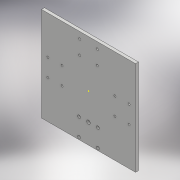
# Autodesk Inventor part: 内层板
Saved by Autodesk Inventor 2017 (Build 210142000, 142)
## iProperties
Part Number: 内层板
Material: 常规
Document SubType Name: 钣金
Designer: PANDA
Density: 1 g/cm^3
Sheet Metal Rule: 默认_mm
Appearance: 默认
Author: PANDA
Autodesk Inventor part; units mm, degrees
ref_plane "YZ Plane" through (0, 0, 0) normal (1, 0, 0) x (0, 1, 0)
ref_plane "XZ Plane" through (0, 0, 0) normal (0, 1, 0) x (-1, 0, 0)
ref_plane "XY Plane" through (0, 0, 0) normal (0, 0, 1) x (1, 0, 0)
sketch "草图19" plane through (0, 0, 0) normal (0, 1, 0) x (-1, 0, 0)
  line L0 (-80, 80) -> (80, 80)
  line L1 (80, 80) -> (80, -80)
  line L2 (80, -80) -> (-80, -80)
  line L3 (-80, -80) -> (-80, 80)
  point P0 (0, 0)
  dimension "d55" = 160
  dimension "d56" = 160
  constraints: 8 end point, 2 parallel, 1 horizontal, 1 perpendicular
  measures "d55" distance of L1.end L2.end
  measures "d56" distance of L0.end L1.end
extrude "拉伸19" add sketch "草图19" along normal blind 5
sketch "草图20" plane through (0, 5, 0) normal (0, 1, 0) x (1, 0, 0)
  circle A0 centre (15, -69) radius 1.8
  point P0 (0, 0)
  dimension "d59" = 3.6
  constraints: 1 centre point
  measures "d59" diameter of A0
extrude "拉伸20" cut sketch "草图20" against normal through all
sketch "草图21" plane through (0, 0, 0) normal (0, -1, 0) x (1, 0, 0)
  circle A0 centre (-15, 69) radius 1.8
  point P0 (0, 0)
  dimension "d62" = 3.6
  constraints: 1 centre point
  measures "d62" diameter of A0
extrude "拉伸21" cut sketch "草图21" against normal through all
sketch "草图26" plane through (0, 0, 0) normal (0, -1, 0) x (1, 0, 0)
  circle A0 centre (15, 45) radius 1.8
  point P0 (0, 0)
  dimension "d73" = 3.6
  constraints: 1 centre point
  measures "d73" diameter of A0
extrude "拉伸24" cut sketch "草图26" against normal through all
sketch "草图27" plane through (0, 0, 0) normal (0, -1, 0) x (1, 0, 0)
  circle A0 centre (-15, 45) radius 1.8
  point P0 (0, 0)
  dimension "d76" = 3.6
  constraints: 1 centre point
  measures "d76" diameter of A0
extrude "拉伸25" cut sketch "草图27" against normal through all
sketch "草图28" plane through (0, 0, 0) normal (0, -1, 0) x (1, 0, 0)
  circle A0 centre (45, 15) radius 1.8
  point P0 (0, 0)
  dimension "d79" = 3.6
  constraints: 1 centre point
  measures "d79" diameter of A0
extrude "拉伸26" cut sketch "草图28" against normal through all
sketch "草图29" plane through (0, 0, 0) normal (0, -1, 0) x (1, 0, 0)
  circle A0 centre (45, -15) radius 1.8
  point P0 (0, 0)
  dimension "d82" = 3.6
  constraints: 1 centre point
  measures "d82" diameter of A0
extrude "拉伸27" cut sketch "草图29" against normal through all
sketch "草图30" plane through (0, 0, 0) normal (0, -1, 0) x (1, 0, 0)
  circle A0 centre (69, 15) radius 1.8
  point P0 (0, 0)
  dimension "d85" = 3.6
  constraints: 1 centre point
  measures "d85" diameter of A0
extrude "拉伸28" cut sketch "草图30" against normal through all
sketch "草图31" plane through (0, 0, 0) normal (0, -1, 0) x (1, 0, 0)
  circle A0 centre (69, -15) radius 1.8
  point P0 (0, 0)
  dimension "d88" = 3.6
  constraints: 1 centre point
  measures "d88" diameter of A0
extrude "拉伸29" cut sketch "草图31" against normal through all
sketch "草图32" plane through (0, 0, 0) normal (0, -1, 0) x (1, 0, 0)
  circle A0 centre (-69, 15) radius 1.8
  point P0 (0, 0)
  dimension "d91" = 3.6
  constraints: 1 centre point
  measures "d91" diameter of A0
extrude "拉伸30" cut sketch "草图32" against normal through all
sketch "草图33" plane through (0, 0, 0) normal (0, -1, 0) x (1, 0, 0)
  circle A0 centre (-45, 15) radius 1.8
  point P0 (0, 0)
  dimension "d94" = 3.6
  constraints: 1 centre point
  measures "d94" diameter of A0
extrude "拉伸31" cut sketch "草图33" against normal through all
sketch "草图34" plane through (0, 0, 0) normal (0, -1, 0) x (1, 0, 0)
  circle A0 centre (-69, -15) radius 1.8
  point P0 (0, 0)
  dimension "d97" = 3.6
  constraints: 1 centre point
  measures "d97" diameter of A0
extrude "拉伸32" cut sketch "草图34" against normal through all
sketch "草图35" plane through (0, 0, 0) normal (0, -1, 0) x (1, 0, 0)
  circle A0 centre (-45, -15) radius 1.8
  point P0 (0, 0)
  dimension "d100" = 3.6
  constraints: 1 centre point
  measures "d100" diameter of A0
extrude "拉伸33" cut sketch "草图35" against normal through all
sketch "草图36" plane through (0, 0, 0) normal (0, -1, 0) x (1, 0, 0)
  point P0 (0, 0)
sketch "草图37" plane through (0, 0, 0) normal (0, -1, 0) x (1, 0, 0)
  circle A0 centre (0, -46) radius 3
  point P0 (0, 0)
  dimension "d103" = 6
  constraints: 1 centre point
  measures "d103" diameter of A0
extrude "拉伸34" cut sketch "草图37" against normal through all
sketch "草图38" plane through (0, 0, 0) normal (0, -1, 0) x (1, 0, 0)
  circle A0 centre (-16, -46) radius 2.5
  point P0 (0, 0)
  dimension "d106" = 5
  constraints: 1 centre point
  measures "d106" diameter of A0
extrude "拉伸35" cut sketch "草图38" against normal through all
sketch "草图39" plane through (0, 0, 0) normal (0, -1, 0) x (1, 0, 0)
  circle A0 centre (16, -46) radius 2.5
  point P0 (0, 0)
  dimension "d109" = 5
  constraints: 1 centre point
  measures "d109" diameter of A0
extrude "拉伸36" cut sketch "草图39" against normal through all
sketch "草图40" plane through (0, 0, 0) normal (0, -1, 0) x (1, 0, 0)
  circle A0 centre (-16, -76) radius 2.5
  point P0 (0, 0)
  dimension "d112" = 5
  constraints: 1 centre point
  measures "d112" diameter of A0
extrude "拉伸37" cut sketch "草图40" against normal through all
sketch "草图41" plane through (0, 0, 0) normal (0, -1, 0) x (1, 0, 0)
  circle A0 centre (16, -76) radius 2.5
  point P0 (0, 0)
  dimension "d115" = 5
  constraints: 1 centre point
  measures "d115" diameter of A0
extrude "拉伸38" cut sketch "草图41" against normal through all
sketch "草图42" plane through (0, 0, 0) normal (0, -1, 0) x (1, 0, 0)
  point P0 (0, 0)
equation "\"折弯半径\" = 厚度"
equation "\"折弯释压宽度\" = 厚度"
equation "\"折弯释压深度\" = 0.5 * 厚度"
equation "\"拐角释压尺寸\" = 4 * 厚度"
equation "\"最小余量\" = 2 * 厚度"
equation "\"过渡半径\" = 折弯半径"
equation "\"Jacobi半径尺寸\" = 折弯半径"
equation "\"间隙大小\" = 厚度"
equation "\"厚度\" = 0.5"
